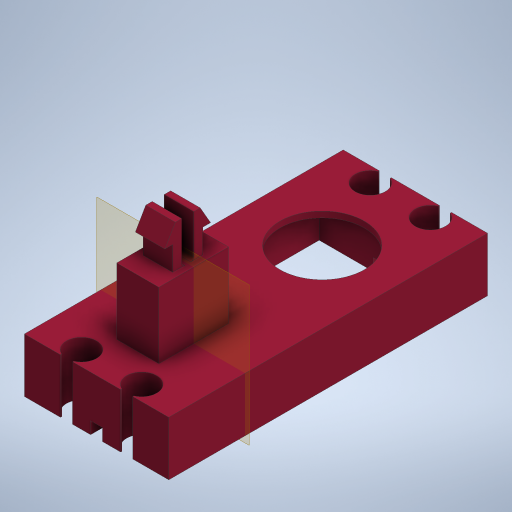
# Autodesk Inventor part: NewServoPlug2
Saved by Autodesk Inventor 2023 (Build 270158000, 158)
## iProperties
Created: 2024-02-07
Part Number: NewServoPlug2
Material: Generic
Document SubType Name: Modeling
Designer: Admin
Density: 1 g/cm^3
Appearance: Default
Author: Admin
Autodesk Inventor part; units mm, degrees
ref_plane "YZ Plane" through (0, 0, 0) normal (1, 0, 0) x (0, 1, 0)
ref_plane "XZ Plane" through (0, 0, 0) normal (0, 1, 0) x (-1, 0, 0)
ref_plane "XY Plane" through (0, 0, 0) normal (0, 0, 1) x (1, 0, 0)
sketch "Sketch1" plane through (0, 0, 0) normal (0, 1, 0) x (-1, 0, 0)
  line L0 (0, 0) -> (20, 0)
  line L1 (20, 0) -> (20, -53) construction
  line L2 (20, -53) -> (0, -53)
  line L3 (0, -53) -> (0, 0) construction
  line L4 (20, -2.5) -> (0, -2.5) construction
  line L5 (10, -50.5) -> (10, -2.5) construction
  line L6 (10, -50.5) -> (10, -53) construction
  line L7 (10, 0) -> (10, -2.5) construction
  circle A0 centre (5, -50.5) radius 2.5
  line L8 (20, -50.5) -> (0, -50.5) construction
  line L9 (5, -50.5) -> (5, -53) construction
  line L10 (6, -52.7913) -> (6, -53)
  line L11 (4, -52.7913) -> (4, -53)
  line L12 (4, -52.7913) -> (5, -52.7913) construction
  line L13 (5, -52.7913) -> (6, -52.7913) construction
  line L14 (20, -26.5) -> (0, -26.5) construction
  circle A1 centre (15, -50.5) radius 2.5
  line L15 (14, -52.7913) -> (14, -53)
  line L16 (16, -52.7913) -> (16, -53)
  circle A2 centre (5, -2.5) radius 2.5
  circle A3 centre (15, -2.5) radius 2.5
  line L17 (14, -0.2087) -> (14, 0)
  line L18 (16, -0.2087) -> (16, 0)
  line L19 (6, -0.2087) -> (6, 0)
  line L20 (4, -0.2087) -> (4, 0)
  line L21 (22, 0) -> (-2, 0)
  line L22 (-2, 0) -> (-2, -53)
  line L23 (-2, -53) -> (22, -53)
  line L24 (22, -53) -> (22, 0)
  line L25 (20, -26.5) -> (22, -26.5) construction
  line L26 (0, -26.5) -> (-2, -26.5) construction
  circle A4 centre (10, -37.5) radius 7
  point P0 (0, -53)
  point P1 (14, -53)
  point P2 (16, 0)
  point P3 (14, 0)
  point P4 (6, 0)
  point P5 (4, 0)
  dimension "d0" = 20
  dimension "d1" = 53
  dimension "d2" = 2.5
  dimension "d3" = 5
  dimension "d4" = 1
  dimension "d5" = 2
  dimension "d6" = 15.5
  dimension "d7" = 14
  constraints: 54 end point, 15 symmetric about line, 11 point on line, 9 midpoint, 9 point on circle, 8 perpendicular, 7 collinear, 5 centre point, 4 parallel, 2 horizontal, 1 tangent, 3 other
  measures "d0" distance between parallel lines of L3 L1
  measures "d1" distance between parallel lines of L2 L0
  measures "d2" distance between parallel lines of L4 L0
  measures "d3" distance from line of L5 L9.start
  measures "d4" distance of L12.end L10.start
  measures "d5" distance between parallel lines of L24 L1
  measures "d6" distance from line of L2 A4.centre
  measures "d7" diameter of A4
extrude "Extrusion1" add sketch "Sketch1" along normal blind 1 contours L0 L20 A2 L19 L17 A3 L18 L21 L24 L23 L2 L16 A1 L15 L10 A0 L11 L22
sketch "Sketch2" plane through (0, 0, 0) normal (0, -1, 0) x (1, 0, 0)
  line L0 (2, 0) -> (2, -53) projected
  line L1 (-22, -53) -> (-22, 0) projected
  line L2 (2, 0) -> (-22, 0)
  line L3 (-22, 0) -> (-22, -53)
  line L4 (2, -53) -> (2, 0)
  arc A0 (-14, -52.7913) -> (-16, -52.7913) centre (-15, -50.5) ccw projected
  arc A1 (-14, -52.7913) -> (-16, -52.7913) centre (-15, -50.5) ccw
  line L5 (-14, -53) -> (-14, -52.7913) projected
  line L6 (-14, -52.7913) -> (-14, -53)
  line L7 (-16, -53) -> (-22, -53) projected
  line L8 (-14, -53) -> (-16, -53)
  line L9 (-16, -52.7913) -> (-16, -53) projected
  line L10 (-16, -53) -> (-16, -52.7913)
  line L11 (-22, -53) -> (-14.5, -53)
  line L12 (-14, -53) -> (2, -53)
  arc A2 (-4, -52.7913) -> (-6, -52.7913) centre (-5, -50.5) ccw projected
  arc A3 (-4, -52.7913) -> (-6, -52.7913) centre (-5, -50.5) ccw
  line L13 (2, -53) -> (-4, -53) projected
  line L14 (-4, -52.7913) -> (-4, -53)
  line L15 (-4, -53) -> (-6, -53)
  line L16 (-6, -53) -> (-6, -52.7913)
  arc A4 (-6, -0.2087) -> (-4, -0.2087) centre (-5, -2.5) ccw projected
  arc A5 (-6, -0.2087) -> (-4, -0.2087) centre (-5, -2.5) ccw
  line L17 (-4, -0.2087) -> (-4, 0) projected
  line L18 (-4, -0.2087) -> (-4, 0)
  line L19 (-14, 0) -> (-6, 0) projected
  line L20 (-4, 0) -> (-6, 0)
  arc A6 (-6, -0.2087) -> (-4, -0.2087) centre (-5, -2.5) ccw projected
  line L21 (-6, 0) -> (-6, -0.2087)
  arc A7 (-16, -0.2087) -> (-14, -0.2087) centre (-15, -2.5) ccw projected
  arc A8 (-16, -0.2087) -> (-14, -0.2087) centre (-15, -2.5) ccw
  line L22 (-14, -0.2087) -> (-14, 0)
  line L23 (-16, 0) -> (-16, -0.2087) projected
  line L24 (-16, 0) -> (-16, -0.2087)
  line L25 (2, 0) -> (2, -53) projected
  line L26 (2, 0) -> (0, 0)
  line L27 (0, 0) -> (0, -53)
  line L28 (0, -53) -> (2, -53)
  line L29 (2, -53) -> (2, 0)
  line L30 (-22, 0) -> (-20, 0)
  line L31 (-20, 0) -> (-20, -53)
  line L32 (-20, -53) -> (-22, -53)
  line L33 (-22, -53) -> (-22, 0)
  line L34 (0, -26.5) -> (2, -26.5) construction
  line L35 (-20, -26.5) -> (-22, -26.5) construction
  line L36 (-20, -6) -> (0, -6)
  line L37 (-20, -47) -> (0, -47)
  line L38 (-10, -47) -> (-10, -53) construction
  line L39 (-6, -53) -> (-14, -53) projected
  line L40 (-10, -6) -> (-10, 0) construction
  point P0 (0, 0)
  point P1 (-22, 0)
  dimension "d10" = 2
  dimension "d11" = 6
  constraints: 60 end point, 11 perpendicular, 10 point on line, 8 midpoint, 8 point on circle, 7 parallel, 4 centre point, 4 coincident, 4 collinear, 3 horizontal, 1 vertical
  measures "d10" distance of L34.start L34.end
  measures "d11" distance between parallel lines of L2 L36
extrude "Extrusion2" add sketch "Sketch2" along normal blind 8 contours L0 L12 L27 L2 | L27 L36 L31 L2 L23 A7 L22 L21 A4 L17 | L12 L14 A2 L16 L5 A0 L9 L7 L31 L37 L27 | L31 L7 L1 L2
sketch "Sketch3" plane through (0, -8, 0) normal (0, -1, 0) x (1, 0, 0)
  line L0 (-10, 0) -> (-10, -53) construction
  line L1 (-6, -53) -> (-14, -53) projected
  line L2 (-11, 0) -> (-9, 0)
  line L3 (-9, 0) -> (-9, -6)
  line L4 (-9, -6) -> (-11, -6)
  line L5 (-11, -6) -> (-11, 0)
  line L6 (-20, -6) -> (0, -6) projected
  line L7 (-6, 0) -> (-14, 0) projected
  line L8 (-11, -53) -> (-9, -53)
  line L9 (-9, -53) -> (-9, -47)
  line L10 (-9, -47) -> (-11, -47)
  line L11 (-11, -47) -> (-11, -53)
  line L12 (0, -47) -> (-20, -47) projected
  line L13 (-14, -53) -> (-6, -53) projected
  point P0 (0, 0)
  point P1 (-10, -6)
  point P2 (-11, -53)
  dimension "d14" = 1
  constraints: 18 end point, 6 collinear, 4 parallel, 2 horizontal, 2 midpoint, 2 perpendicular, 1 point on line
  measures "d14" distance between parallel lines of L0 L5
extrude "Extrusion3" cut sketch "Sketch3" against normal blind 2
sketch "Sketch4" plane through (0, 1, 0) normal (0, 1, 0) x (1, 0, 0)
  line L0 (-12.45, 23.9) -> (-7.55, 23.9) construction
  line L1 (-7.55, 23.9) -> (-7.55, 31.5) construction
  line L2 (-7.55, 31.5) -> (-12.45, 31.5) construction
  line L3 (-12.45, 31.5) -> (-12.45, 23.9) construction
  circle A0 centre (-10, 37.5) radius 7 projected
  line L4 (-10, 31.5) -> (-10, 37.5) construction
  line L5 (-12.45, 27.7) -> (-7.55, 27.7) construction
  line L6 (-12.45, 16.5) -> (-7.55, 16.5)
  line L7 (-7.55, 16.5) -> (-7.55, 8.9)
  line L8 (-7.55, 8.9) -> (-12.45, 8.9)
  line L9 (-12.45, 8.9) -> (-12.45, 16.5)
  line L10 (-12.45, 12.7) -> (-7.55, 12.7) construction
  point P0 (0, 0)
  point P1 (-10, 27.7)
  dimension "d17" = 9.8
  dimension "d18" = 15
  dimension "d19" = 7.6
  dimension "d20" = 4.9
  constraints: 22 end point, 6 midpoint, 4 parallel, 3 collinear, 2 horizontal, 2 perpendicular, 1 vertical
  measures "d17" distance of L4.end point (-10, 27.7)
  measures "d18" distance between parallel lines of L5 L10
  measures "d19" distance between parallel lines of L0 L2
  measures "d20" distance between parallel lines of L3 L1
extrude "Extrusion4" add sketch "Sketch4" along normal blind 18 contours L6 L7 L8 L9
ref_plane "Work Plane1" through (-12.45, 1, -12.7) normal (0, 0, 1) x (1, 0, 0)
sketch "Sketch5" plane through (-7.55, 1, -8.9) normal (1, 0, 0) x (0, 0, -1)
  line L0 (7.6, 0) -> (7.6, 18)
  line L1 (7.6, 11) -> (0, 11)
  line L2 (0, 18) -> (7.6, 18)
  line L3 (2.8, 11) -> (2.8, 18)
  line L4 (7.6, 18) -> (0, 18)
  line L5 (1.7321, 18) -> (0, 15)
  line L6 (0, 15) -> (1.3, 15)
  line L7 (0, 0) -> (0, 18)
  line L8 (1.3, 15) -> (1.3, 11)
  line L9 (3.8, 11) -> (3.8, 18) construction
  line L10 (2.8, 18) -> (1.7321, 18)
  line L11 (0, 0) -> (0, 18)
  line L12 (1.7321, 18) -> (0, 18)
  line L13 (0, 18) -> (0, 15)
  line L14 (0, 11) -> (0, 15)
  line L15 (3.8, 11) -> (3.8, 18)
  line L16 (2.8, 18) -> (3.8, 18)
  line L17 (7.6, 0) -> (7.6, 18) projected
  line L18 (0, 0) -> (0, 18) projected
  line L19 (0, 18) -> (7.6, 18) projected
  point P0 (-8.9, -1)
  dimension "d23" = 7
  dimension "d24" = 1
  dimension "d25" = 4
  dimension "d26" = 60
  dimension "d27" = 1.5
  constraints: 34 end point, 7 collinear, 6 point on line, 4 perpendicular, 2 midpoint, 2 vertical, 1 horizontal
  measures "d23" distance between parallel lines of L2 L1
  measures "d24" distance between parallel lines of L9 L3
  measures "d25" distance between parallel lines of L1 L6
  measures "d26" angle of L6 L5
  measures "d27" distance between parallel lines of L8 L3
extrude "Extrusion5" cut sketch "Sketch5" against normal up to surface (4.9 mm away) contours L1 L3 L2 L15 | L1 L7 L6 L8 | L5 L7 L2
mirror "Mirror1" about plane through (-12.45, 1, -12.7) normal (0, 0, 1) of "Extrusion5"
sketch "Sketch6" plane through (-7.55, 1, -8.9) normal (1, 0, 0) x (0, 0, -1)
  line L0 (44.1, 0) -> (-8.9, 0) projected
  line L1 (9.6, 11) -> (-2, 11)
  line L2 (-2, 11) -> (-2, 0)
  line L3 (-2, 0) -> (9.6, 0)
  line L4 (9.6, 0) -> (9.6, 11)
  line L5 (3.8, 11) -> (3.8, 0) construction
  line L6 (2.8, 11) -> (4.8, 11) projected
  line L7 (7.6, 11) -> (6.3, 11) projected
  line L8 (7.6, 0) -> (7.6, 11) projected
  point P0 (-8.9, -1)
  point P1 (9.6, 0)
  dimension "d30" = 2
  constraints: 10 end point, 3 midpoint, 2 parallel, 2 point on line, 1 collinear, 1 horizontal, 1 perpendicular
  measures "d30" distance between parallel lines of L4 L8
extrude "Extrusion6" add sketch "Sketch6" along normal blind 1 and the other way blind 6
fillet "Fillet1" radius 0.5 2 edges at (-10, 12, -11.7) (-10, 12, -13.7)
body "Solid1"
